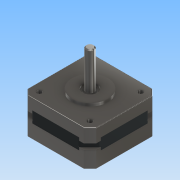
# Autodesk Inventor part: Мотор
Saved by Autodesk Inventor 2017 (Build 210142000, 142)
## iProperties
Part Number: Мотор
Material: Типовые
Document SubType Name: Modeling
Designer: STALKER
Density: 1 g/cm^3
Appearance: Сталь — полированная
Author: STALKER
Autodesk Inventor part; units mm, degrees
ref_plane "YZ Plane" through (0, 0, 0) normal (1, 0, 0) x (0, 1, 0)
ref_plane "XZ Plane" through (0, 0, 0) normal (0, 1, 0) x (-1, 0, 0)
sketch "Эскиз1" plane through (0, 0, 0) normal (0, 0, 1) x (1, 0, 0)
  line L0 (21, -21) -> (-21, -21)
  line L1 (-21, -21) -> (-21, 21)
  line L2 (-21, 21) -> (21, 21)
  line L3 (21, 21) -> (21, -21)
  line L4 (21, -21) -> (-21, 21) construction
  line L5 (-21, -21) -> (21, 21) construction
  line L6 (15.5, 15.5) -> (-15.5, 15.5) construction
  line L7 (-15.5, 15.5) -> (-15.5, -15.5) construction
  line L8 (-15.5, -15.5) -> (15.5, -15.5) construction
  line L9 (15.5, -15.5) -> (15.5, 15.5) construction
  line L10 (15.5, 15.5) -> (-15.5, -15.5) construction
  line L11 (-15.5, 15.5) -> (15.5, -15.5) construction
  circle A0 centre (0, 0) radius 2.5
  circle A1 centre (0, 0) radius 4.5
  circle A2 centre (0, 0) radius 11
  circle A3 centre (0, 0) radius 3.5
  circle A4 centre (15.5, 15.5) radius 1.5
  circle A5 centre (-15.5, 15.5) radius 1.5
  circle A6 centre (15.5, -15.5) radius 1.5
  circle A7 centre (-15.5, -15.5) radius 1.5
  circle A8 centre (15.5, 15.5) radius 3
  circle A9 centre (-15.5, 15.5) radius 3
  circle A10 centre (15.5, -15.5) radius 3
  circle A11 centre (-15.5, -15.5) radius 3
  line L12 (21, 17.1838) -> (17.1838, 21)
  line L13 (-17.1838, 21) -> (-21, 17.1838)
  line L14 (21, -17.184) -> (17.184, -21)
  line L15 (-17.184, -21) -> (-21, -17.184)
  line L16 (0, 0) -> (0, 33) construction
  line L17 (0, 0) -> (-47, 0) construction
  dimension "d0" = 42
  dimension "d1" = 42
  dimension "d2" = 31
  dimension "d3" = 31
  dimension "d4" = 5
  dimension "d9" = 9
  dimension "d10" = 22
  dimension "d15" = 7
  dimension "d24" = 3
  dimension "d25" = 3
  dimension "d26" = 3
  dimension "d27" = 3
  dimension "d30" = 6
  dimension "d31" = 6
  dimension "d32" = 6
  dimension "d33" = 6
  dimension "d41" = 45
  dimension "d42" = 45
  dimension "d43" = 27
  dimension "d44" = 3.8162
  dimension "d45" = 3.8162
  dimension "d46" = 3.816
  dimension "d47" = 27.0002
  dimension "d48" = 3.816
  constraints: 36 end point, 12 centre point, 11 coincident, 9 point on line, 6 perpendicular, 4 midpoint, 4 parallel, 3 horizontal, 1 vertical, 1 other
  measures "d0" distance of L1.end L2.end
  measures "d1" distance of L0.end L1.end
  measures "d2" distance of L8.end L7.end
  measures "d3" distance of L7.end L6.end
  measures "d4" diameter of A0
  measures "d9" diameter of A1
  measures "d10" diameter of A2
  measures "d15" diameter of A3
  measures "d24" diameter of A4
  measures "d25" diameter of A5
  measures "d26" diameter of A6
  measures "d27" diameter of A7
  measures "d30" diameter of A8
  measures "d31" diameter of A9
  measures "d32" diameter of A10
  measures "d33" diameter of A11
  measures "d41" angle of L3 L12
  measures "d42" angle of L0 L15
  measures "d43" distance from line of A1.centre L12
  measures "d44" distance from line of L3 L12.end
  measures "d45" distance from line of L1 L13.start
  measures "d46" distance from line of L0 L15.end
  measures "d47" distance from line of L16.start L15
  measures "d48" distance of L0.start L14.end
extrude "Выдавливание1" add sketch "Эскиз1" along normal blind 46 contours A0
extrude "Выдавливание2" cut sketch "Эскиз1" along normal blind 1.4 contours A0
extrude "Выдавливание3" add sketch "Эскиз1" along normal blind 23.8 contours A2
extrude "Выдавливание4" add sketch "Эскиз1" along normal blind 22 contours L0 L14 L3 | L0 L15 L1 L13 L2 L12 L3 L14 | L0 L1 L15 | L12 L2 L3 | L1 L2 L13 | A4 | A5 | A6 | A7 | A8 | A9 | A10 | A11
extrude "Выдавливание5" add sketch "Эскиз1" along normal blind 23 contours A3
extrude "Выдавливание6" cut sketch "Эскиз1" along normal blind 2 contours A3
extrude "Выдавливание7" add sketch "Эскиз1" along normal blind 22.8 contours A1
extrude "Выдавливание8" cut sketch "Эскиз1" along normal blind 2.5 contours A1
extrude "Выдавливание9" cut sketch "Эскиз1" along normal blind 30 contours A4 | A5 | A6 | A7
extrude "Выдавливание10" cut sketch "Эскиз1" along normal blind 2.5 contours A8 | A9 | A10 | A11
extrude "Выдавливание11" cut sketch "Эскиз1" along normal blind 40 contours L0 L14 L3 | L0 L1 L15 | L12 L2 L3 | L1 L2 L13
ref_plane "РабПлоскость1" through (0, 0, 12) normal (0, 0, -1) x (-1, 0, 0)
sketch "Эскиз2" plane through (0, 0, 12) normal (0, 0, -1) x (-1, 0, 0)
  line L0 (14.4553, 20.9) -> (-14.4553, 20.9)
  line L1 (-20.9, 14.4553) -> (-20.9, -14.4553)
  line L2 (-14.4553, -20.9) -> (14.4553, -20.9)
  line L3 (20.9, -14.4553) -> (20.9, 14.4553)
  line L4 (20.9, 20.9) -> (-20.9, -20.9) construction
  line L5 (-20.9, 20.9) -> (20.9, -20.9) construction
  line L6 (-14.4553, -20.9) -> (-20.9, -14.4553)
  line L7 (14.4553, 20.9) -> (20.9, 14.4553)
  line L8 (14.4553, -20.9) -> (21, -14.3553)
  line L9 (-20.9, 14.4553) -> (-14.4553, 20.9)
  line L10 (38, 38) -> (-38, 38)
  line L11 (-38, 38) -> (-38, -38)
  line L12 (-38, -38) -> (38, -38)
  line L13 (38, -38) -> (38, 38)
  line L14 (38, 38) -> (-38, -38) construction
  line L15 (-38, 38) -> (38, -38) construction
  line L16 (-20.9, -14.4553) -> (-21, -14.3553)
  line L17 (-21, -14.3553) -> (-21, 14.3553)
  line L18 (-21, 14.3553) -> (-20.9, 14.4553)
  line L19 (-14.4553, 20.9) -> (-14.3553, 21)
  line L20 (-14.3553, 21) -> (14.3553, 21)
  line L21 (14.3553, 21) -> (14.4553, 20.9)
  line L22 (20.9, 14.4553) -> (21, 14.3553)
  line L23 (21, 14.3553) -> (21, -14.3553)
  line L24 (14.4553, -20.9) -> (14.3553, -21)
  line L25 (14.3553, -21) -> (-14.3553, -21)
  line L26 (-14.4553, -20.9) -> (-14.3553, -21)
  point P0 (0, 0)
  dimension "d52" = 41.8
  dimension "d53" = 41.8
  dimension "d54" = 45
  dimension "d55" = 45
  dimension "d56" = 45
  dimension "d57" = 45
  dimension "d58" = 25
  dimension "d59" = 25
  dimension "d60" = 25
  dimension "d61" = 25
  constraints: 54 end point, 8 parallel, 4 midpoint, 4 point on line, 3 perpendicular, 2 collinear, 2 horizontal
  measures "d52" distance between parallel lines of L3 L1
  measures "d53" distance between parallel lines of L0 L2
  measures "d54" angle of L2 L6
  measures "d55" angle of L0 L7
  measures "d56" angle of L3 L8
  measures "d57" angle of L0 L9
  measures "d58" distance from line of L6 point (0, 0)
  measures "d59" distance from line of L7 point (0, 0)
  measures "d60" distance from line of L9 point (0, 0)
  measures "d61" distance from line of point (0, 0) L8
extrude "Выдавливание12" cut sketch "Эскиз2" along normal mid plane 3.5
extrude "Выдавливание13" cut sketch "Эскиз2" along normal mid plane 7 contours L0 L19 L20 L21 | L22 L23 L8 L3 | L1 L16 L17 L18 | L24 L25 L26 L2
fillet "Сопряжение1" radius 2 8 edges at (14.4553, -20.9, 12) (20.9, -14.4553, 12) (-14.4553, -20.9, 12) (-20.9, -14.4553, 12) (-20.9, 14.4553, 12) (-14.4553, 20.9, 12) (14.4553, 20.9, 12) (20.9, 14.4553, 12)
fillet "Сопряжение2" radius 0.5 16 edges at (21, -0.0001, 22) (19.092, -19.092, 22) (0, -21, 22) (-19.092, -19.092, 22) (-21, -0.0001, 22) (-19.0919, 19.0919, 22) (0, 21, 22) (19.0919, 19.0919, 22) (0, -21, 0) (19.092, -19.092, 0) (21, -0.0001, 0) (19.0919, 19.0919, 0) (0, 21, 0) (-19.0919, 19.0919, 0) (-21, -0.0001, 0) (-19.092, -19.092, 0)
fillet "Сопряжение3" radius 0.3 1 edges at (-4.5, 0, 0)
fillet "Сопряжение4" radius 0.3 4 edges at (12.5, -15.5, 0) (-18.5, -15.5, 0) (-18.5, 15.5, 0) (12.5, 15.5, 0)
chamfer "Фаска1" distance 0.6 angle 45 1 edges at (-2.5, 0, 46)
